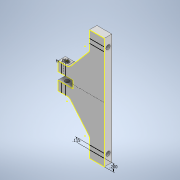
# Autodesk Inventor part: mount 3D print
Saved by Autodesk Inventor 2020.1 (Build 241239000, 239)
## iProperties
Created: 2019-10-24
Part Number: mount 3D print
Material: Generic
Document SubType Name: Modeling
Designer: amirs
Density: 1 g/cm^3
Appearance: Default
Author: amirs
Autodesk Inventor part; units mm, degrees
ref_plane "YZ Plane" through (0, 0, 0) normal (1, 0, 0) x (0, 1, 0)
ref_plane "XZ Plane" through (0, 0, 0) normal (0, 1, 0) x (-1, 0, 0)
sketch "Sketch1" plane through (0, 0, 0) normal (0, 0, 1) x (1, 0, 0)
  line L0 (0, 0) -> (0, 76.2)
  line L1 (0, 76.2) -> (-10.16, 76.2)
  line L2 (-10.16, 76.2) -> (-10.16, 63.5)
  line L3 (-10.16, 63.5) -> (-24.13, 46.99)
  line L4 (-24.13, 46.99) -> (-31.75, 46.99)
  line L5 (-31.75, 46.99) -> (-31.75, 40.64)
  line L6 (-21.59, 35.56) -> (-31.75, 35.56)
  line L7 (-31.75, 35.56) -> (-31.75, 29.21)
  line L8 (-31.75, 29.21) -> (-24.13, 29.21)
  line L9 (-24.13, 29.21) -> (-10.16, 12.7)
  line L10 (-10.16, 12.7) -> (-10.16, 0)
  line L11 (-10.16, 0) -> (0, 0)
  line L12 (-31.75, 40.64) -> (-21.59, 40.64)
  line L13 (-21.59, 40.64) -> (-21.59, 35.56)
  line L14 (-21.59, 38.1) -> (-22.098, 38.1) construction
  dimension "d1" = 10.16
  dimension "d2" = 31.75
  dimension "d3" = 76.2
  dimension "d5" = 7.62
  dimension "d8" = 5.08
  dimension "d11" = 38.1
  dimension "d12" = 6.35
  dimension "d14" = 12.7
  dimension "d23" = 10.16
  constraints: 30 end point, 6 perpendicular, 4 point on line, 3 equal length, 3 horizontal, 1 midpoint, 1 parallel, 1 vertical
  measures "d1" distance of L0.end L1.end
  measures "d2" distance between parallel lines of L0 L5
  measures "d3" distance of L0.start L0.end
  measures "d5" distance of L7.end L8.end
  measures "d8" distance of L12.end L6.start
  measures "d11" distance between parallel lines of L11 L14
  measures "d12" distance of L6.end L7.end
  measures "d14" distance of L1.end L2.end
  measures "d23" distance between parallel lines of L7 L13
extrude "Extrusion1" add sketch "Sketch1" along normal blind 5.08
fillet "Fillet1" radius 3.175 4 edges at (-10.16, 12.7, 2.54) (-24.13, 29.21, 2.54) (-10.16, 63.5, 2.54) (-24.13, 46.99, 2.54)
sketch "Sketch2" plane through (0, 0, 5.08) normal (0, 0, 1) x (1, 0, 0)
  line L0 (-10.16, 11.537) -> (-10.16, 0) projected
  line L1 (-10.16, 0) -> (0, 0) projected
  line L2 (0, 0) -> (0, 76.2) projected
  line L3 (0, 76.2) -> (-10.16, 76.2) projected
  line L4 (-10.16, 76.2) -> (-10.16, 64.663) projected
  line L5 (-10.9112, 62.6122) -> (-23.1788, 48.1141) projected
  line L6 (-25.6026, 46.99) -> (-31.75, 46.99) projected
  line L7 (-31.75, 46.99) -> (-31.75, 40.64) projected
  line L8 (-31.75, 40.64) -> (-21.59, 40.64) projected
  line L9 (-21.59, 40.64) -> (-21.59, 35.56) projected
  line L10 (-21.59, 35.56) -> (-31.75, 35.56) projected
  line L11 (-31.75, 35.56) -> (-31.75, 29.21) projected
  line L12 (-31.75, 29.21) -> (-25.6026, 29.21) projected
  line L13 (-23.1788, 28.0859) -> (-10.9112, 13.5878) projected
  line L14 (-24.13, 46.99) -> (-31.75, 46.99) construction
  line L15 (-27.94, 46.99) -> (-27.94, 40.64) construction
  line L16 (-31.75, 40.64) -> (-21.59, 40.64) construction
  line L17 (-29.4005, 46.99) -> (-29.4005, 40.64)
  line L18 (-26.4795, 46.99) -> (-26.4795, 40.64)
  line L19 (0, 0) -> (0, 76.2) construction
  line L20 (0, 38.1) -> (-22.098, 38.1) construction
  line L21 (-29.4005, 29.21) -> (-29.4005, 35.56)
  line L22 (-26.4795, 29.21) -> (-26.4795, 35.56)
  line L23 (-10.16, 12.7) -> (-10.16, 0) projected
  line L24 (-10.16, 5.08) -> (0, 5.08)
  line L25 (-10.16, 8.001) -> (0, 8.001)
  line L26 (-10.16, 71.12) -> (0, 71.12)
  line L27 (-10.16, 68.199) -> (0, 68.199)
  arc A0 (-23.1788, 28.0859) -> (-25.6026, 29.21) centre (-25.6026, 26.035) ccw projected
  arc A1 (-10.16, 11.537) -> (-10.9112, 13.5878) centre (-13.335, 11.537) ccw projected
  arc A2 (-10.9112, 62.6122) -> (-10.16, 64.663) centre (-13.335, 64.663) ccw projected
  arc A3 (-25.6026, 46.99) -> (-23.1788, 48.1141) centre (-25.6026, 50.165) ccw projected
  dimension "d18" = 1.4605
  dimension "d19" = 1.4605
  dimension "d21" = 2.921
  dimension "d22" = 5.08
  constraints: 20 end point, 9 point on line, 8 symmetric about line, 2 midpoint, 2 parallel, 2 perpendicular, 1 horizontal, 1 vertical
  measures "d18" distance between parallel lines of L15 L18
  measures "d19" distance between parallel lines of L17 L15
  measures "d21" distance between parallel lines of L24 L25
  measures "d22" distance between parallel lines of L1 L24
sketch "Sketch3" plane through (-31.75, 46.99, 0) normal (0, 1, 0) x (1, 0, 0)
  line L0 (3.81, -5.08) -> (3.81, 0) construction
  circle A0 centre (3.81, -2.54) radius 1.4605
  point P0 (31.75, 0)
  dimension "d24" = 2.921
  constraints: 2 end point, 1 centre point, 1 midpoint, 1 vertical
  measures "d24" diameter of A0
extrude "Extrusion2" cut sketch "Sketch3" against normal blind 25.4
sketch "Sketch4" plane through (-10.16, 0, 0) normal (-1, 0, 0) x (0, 0, 1)
  line L0 (0, 0) -> (0, 76.2) construction
  line L1 (0, 12.7) -> (0, 0) construction
  line L2 (0, 6.5405) -> (5.08, 6.5405) construction
  line L3 (0, 0) -> (5.08, 0) construction
  circle A0 centre (2.54, 6.5405) radius 1.4605
  point P0 (5.08, 5.08)
  dimension "d27" = 6.5405
  dimension "d28" = 2.921
  constraints: 2 end point, 1 centre point, 1 horizontal, 1 midpoint, 1 point on line
  measures "d27" distance between parallel lines of L3 L2
  measures "d28" diameter of A0
extrude "Extrusion3" cut sketch "Sketch4" against normal blind 25.4
ref_plane "Work Plane1" through (0, 38.1, 5.08) normal (0, 1, 0) x (-1, 0, 0)
mirror "Mirror1" about plane through (0, 38.1, 5.08) normal (0, 1, 0) of "Extrusion3"
equation "\"d19\" = d18"
body "Solid1"
